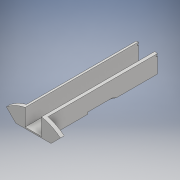
# Autodesk Inventor part: Hull_batt_pillar
Saved by Autodesk Inventor 2018 (Build 220112000, 112)
## iProperties
Created: 2018-05-01
Part Number: Hull_batt_pillar
Material: Generic
Document SubType Name: Modeling
Designer: suchanek
Density: 1 g/cm^3
Appearance: Default
Author: suchanek
Autodesk Inventor part; units mm, degrees
ref_plane "YZ Plane" through (0, 0, 0) normal (1, 0, 0) x (0, 1, 0)
ref_plane "XZ Plane" through (0, 0, 0) normal (0, 1, 0) x (-1, 0, 0)
ref_plane "XY Plane" through (0, 0, 0) normal (0, 0, 1) x (1, 0, 0)
sketch "Sketch1" plane through (0, 0, 0) normal (0, 1, 0) x (-1, 0, 0)
  arc A0 (21.0006, 25.4554) -> (6.35, 32.3833) centre (0, 0) ccw
  line L0 (0, 0) -> (-23.3345, 23.3345)
  line L1 (0, 0) -> (33, 0) construction
  line L2 (0, 0) -> (0, 8.3369)
  line L3 (-23.3345, 23.3345) -> (-9.1924, 9.1924)
  line L4 (-9.1924, 9.1924) -> (-6.965, 11.4198)
  line L5 (-6.965, 11.4198) -> (-13.7089, 18.1636)
  line L6 (-21.1071, 25.5619) -> (-23.3345, 23.3345)
  line L7 (23.3345, 23.3345) -> (9.1924, 9.1924)
  line L8 (9.1924, 9.1924) -> (6.965, 11.4198)
  line L9 (6.965, 11.4198) -> (13.7089, 18.1636)
  line L10 (21.1071, 25.5619) -> (23.3345, 23.3345)
  line L11 (-6.35, 32.3833) -> (6.35, 32.3833)
  line L12 (6.35, 32.3833) -> (6.35, 19.1636)
  line L13 (6.35, 19.1636) -> (-6.35, 19.1636)
  line L14 (-6.35, 19.1636) -> (-6.35, 32.3833)
  line L15 (13.7089, 18.1636) -> (-13.7089, 18.1636)
  line L16 (-13.7089, 18.1636) -> (-21.1071, 25.5619)
  arc A1 (-6.35, 32.3833) -> (-21.0006, 25.4554) centre (0, 0) ccw
  arc A2 (6.35, 32.3833) -> (-6.35, 32.3833) centre (0, 0) ccw
  line L17 (13.7089, 18.1636) -> (21.1071, 25.5619)
  point P0 (-6.35, 31.3636)
  dimension "d0" = 33
  dimension "d1" = 33
  dimension "d2" = 135
  dimension "d3" = 3.15
  dimension "d4" = 20
  dimension "d5" = 32
  dimension "d7" = 12.2
  dimension "d8" = 12.7
  dimension "d33" = 18.1636
  constraints: 36 end point, 7 point on circle, 6 point on line, 5 parallel, 4 symmetric about line, 3 centre point, 3 horizontal, 2 perpendicular, 1 coincident, 1 equal length, 1 vertical
  measures "d0" radius of A0
  measures "d1" distance of L0.start L0.end
  measures "d2" angle of L1 L0
  measures "d3" distance of L4.end L3.end
  measures "d4" distance between parallel lines of L6 L4
  measures "d5" distance of point (0, 0) point (-6.35, 31.364)
  measures "d7" distance of L13.end point (-6.35, 31.364)
  measures "d8" distance of L12.end L13.end
  measures "d33" distance from line of L0.start L15
extrude "Extrusion1" add sketch "Sketch1" along normal blind 3 contours L17 L15 L16 A1 L14 L13 L12 A0
sketch "Sketch2" plane through (0, 3, 0) normal (0, 1, 0) x (1, 0, 0)
  arc A0 (6.35, -32.3833) -> (21.0006, -25.4554) centre (0, 0) ccw projected
  line L0 (8.35, -31.9261) -> (8.35, -18.1636)
  line L1 (13.7089, -18.1636) -> (-13.7089, -18.1636) projected
  line L2 (-8.35, -18.1636) -> (-8.35, -31.9261)
  arc A1 (-21.0006, -25.4554) -> (-6.35, -32.3833) centre (0, 0) ccw projected
  line L3 (-6.35, -19.1636) -> (6.35, -19.1636) projected
  line L4 (6.35, -32.3833) -> (6.35, -19.1636)
  line L5 (6.35, -19.1636) -> (-6.35, -19.1636)
  line L6 (-6.35, -32.3833) -> (-6.35, -19.1636) projected
  line L7 (-6.35, -19.1636) -> (-6.35, -32.3833)
  dimension "d14" = 2
  constraints: 10 end point, 3 vertical, 2 perpendicular, 2 point on circle, 2 point on line, 1 horizontal alignment
  measures "d14" distance between parallel lines of L6 L2
extrude "Extrusion2" add sketch "Sketch2" along normal blind 85
ref_plane "Work Plane1" through (8.35, 3, 18.1636) normal (-0.7071068, 0, -0.7071068) x (0, 1, 0)
sketch "Sketch4" plane through (8.35, 3, 18.1636) normal (-0.7071068, 0, -0.7071068) x (0, 1, 0)
  circle A0 centre (49, 6.9393) radius 8
  line L0 (85, -9.7316) -> (85, 0) projected
  line L1 (-3, 3.7893) -> (0, 3.7893) projected
  line L2 (49, -1.0607) -> (31, -1.0607)
  line L3 (31, -1.0607) -> (31, 14.9393)
  line L4 (31, 14.9393) -> (49, 14.9393)
  line L5 (49, 14.9393) -> (49, -1.0607)
  point P0 (-3, 6.9393)
  dimension "d19" = 16
  dimension "d20" = 36
  dimension "d21" = 3.15
  dimension "d22" = 18
  dimension "d23" = 16
  constraints: 8 end point, 2 parallel, 2 point on circle, 1 centre point, 1 horizontal, 1 perpendicular
  measures "d19" diameter of A0
  measures "d20" distance from line of L0 A0.centre
  measures "d21" distance from line of L1 A0.centre
  measures "d22" distance of L3.end L4.end
  measures "d23" distance of L2.end L3.end
extrude "Extrusion3" cut sketch "Sketch4" along normal through all both and the other way through all
ref_plane "Work Plane3" through (0, 88, 18.1636) normal (-1, 0, 0) x (0, 0, 1)
mirror "Mirror1" about plane through (0, 88, 18.1636) normal (-1, 0, 0) of "Extrusion3"
sketch "Sketch5" plane through (0, 88, 0) normal (0, 1, 0) x (1, 0, 0)
  line L0 (8.35, -30.3833) -> (-8.35, -30.3833)
  line L1 (-8.35, -30.3833) -> (-8.35, -31.3833)
  line L2 (-8.35, -31.3833) -> (8.35, -31.3833)
  line L3 (8.35, -31.3833) -> (8.35, -30.3833)
  line L4 (8.35, -31.9261) -> (8.35, -18.1636) projected
  arc A0 (6.35, -32.3833) -> (21.0006, -25.4554) centre (0, 0) ccw projected
  dimension "d27" = 16.7
  dimension "d28" = 1
  dimension "d29" = 1
  constraints: 8 end point, 2 parallel, 1 collinear, 1 horizontal, 1 perpendicular
  measures "d27" distance of L2.end L1.end
  measures "d28" distance of L1.end L0.end
  measures "d29" distance from line of A0.start L2
extrude "Extrusion4" cut sketch "Sketch5" against normal blind 1.1
fillet "Fillet1" radius 0.5 4 edges at (7.35, 86.9, 31.3833) (-7.35, 86.9, 31.3833) (-7.35, 86.9, 30.3833) (7.35, 86.9, 30.3833)
sketch "Sketch6" plane through (13.7089, 0, 18.1636) normal (0, 0, -1) x (-1, 0, 0)
  line L0 (8.4589, 16) -> (18.9589, 16)
  line L1 (18.9589, 16) -> (18.9589, 54)
  line L2 (18.9589, 54) -> (8.4589, 54)
  line L3 (8.4589, 54) -> (8.4589, 16)
  line L4 (13.7089, 0) -> (13.7089, 8.6013)
  line L5 (5.3589, 88) -> (22.0589, 88) projected
  dimension "d36" = 10.5
  dimension "d37" = 38
  dimension "d38" = 34
  constraints: 10 end point, 2 parallel, 1 horizontal, 1 perpendicular, 1 vertical, 1 other
  measures "d36" distance of L1.end L2.end
  measures "d37" distance of L0.end L1.end
  measures "d38" distance between parallel lines of L5 L2
extrude "Extrusion5" cut sketch "Sketch6" against normal blind 0.336
body "Solid1"
